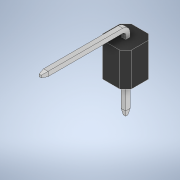
# Autodesk Inventor part: MaleHeaderPin
Saved by Autodesk Inventor 2021 (Build 250183000, 183)
## iProperties
Created: 2020-01-06
Part Number: MaleHeaderPin
Material: Generic
Document SubType Name: Modeling
Designer: ermoz
Density: 1 g/cm^3
Appearance: Default
Mass: 0.0192281 g
Surface Area: 0.622522 cm^2
Volume: 0.0192281 cm^3
Author: ermoz
Autodesk Inventor part; units mm, degrees
ref_plane "YZ Plane" through (0, 0, 0) normal (1, 0, 0) x (0, 1, 0)
ref_plane "XZ Plane" through (0, 0, 0) normal (0, 1, 0) x (-1, 0, 0)
ref_plane "XY Plane" through (0, 0, 0) normal (0, 0, 1) x (1, 0, 0)
sketch "Sketch1" plane through (0, 0, 0) normal (0, 1, 0) x (-1, 0, 0)
  line L0 (-1.27, 1.27) -> (1.27, 1.27)
  line L1 (1.27, 1.27) -> (1.27, -1.27)
  line L2 (1.27, -1.27) -> (-1.27, -1.27)
  line L3 (-1.27, -1.27) -> (-1.27, 1.27)
  line L4 (-1.27, 1.27) -> (1.27, -1.27) construction
  line L5 (1.27, 1.27) -> (-1.27, -1.27) construction
  line L6 (-0.3, 0.3) -> (0.3, 0.3)
  line L7 (0.3, 0.3) -> (0.3, -0.3)
  line L8 (0.3, -0.3) -> (-0.3, -0.3)
  line L9 (-0.3, -0.3) -> (-0.3, 0.3)
  line L10 (-0.3, 0.3) -> (0.3, -0.3) construction
  line L11 (0.3, 0.3) -> (-0.3, -0.3) construction
  point P0 (0, 0)
  dimension "d0" = 2.54
  dimension "d1" = 2.54
  dimension "d2" = 0.6
  dimension "d3" = 0.6
  constraints: 24 end point, 4 midpoint, 4 parallel, 2 horizontal, 2 perpendicular
  measures "d0" distance of L1.end L2.end
  measures "d1" distance of L0.end L1.end
  measures "d2" distance of L7.end L8.end
  measures "d3" distance of L6.end L7.end
extrude "Extrusion1" add sketch "Sketch1" along normal blind 9 and the other way blind 3 contours L6 L7 L8 L9
extrude "Extrusion2" add sketch "Sketch1" along normal blind 3 separate body
sketch "Sketch2" plane through (0, 9, 0) normal (0, 1, 0) x (1, 0, 0)
  line L0 (-0.2, -0.2) -> (0.2, -0.2)
  line L1 (0.2, -0.2) -> (0.2, 0.2)
  line L2 (0.2, 0.2) -> (-0.2, 0.2)
  line L3 (-0.2, 0.2) -> (-0.2, -0.2)
  line L4 (-0.2, -0.2) -> (0.2, 0.2) construction
  line L5 (0.2, -0.2) -> (-0.2, 0.2) construction
  line L6 (-2.0289, -1.4927) -> (2.0289, -1.4927)
  line L7 (2.0289, -1.4927) -> (2.0289, 1.4927)
  line L8 (2.0289, 1.4927) -> (-2.0289, 1.4927)
  line L9 (-2.0289, 1.4927) -> (-2.0289, -1.4927)
  line L10 (-2.0289, -1.4927) -> (2.0289, 1.4927) construction
  line L11 (2.0289, -1.4927) -> (-2.0289, 1.4927) construction
  point P0 (0, 0)
  dimension "d37" = 0.4
  dimension "d38" = 0.4
  constraints: 24 end point, 4 midpoint, 4 parallel, 2 horizontal, 2 perpendicular
  measures "d37" distance of L2.end L1.end
  measures "d38" distance of L1.end L0.end
extrude "Extrusion3" cut sketch "Sketch2" against normal blind 20 bodies 1
sketch "Sketch3" plane through (0, 3, 0) normal (0, 1, 0) x (1, 0, 0)
  line L0 (-0.3, 0.3) -> (0.3, 0.3) projected
  line L1 (-0.3, -0.3) -> (0.3, -0.3)
  line L2 (0.3, -0.3) -> (0.3, 0.3)
  line L3 (0.3, 0.3) -> (-0.3, 0.3)
  line L4 (-0.3, 0.3) -> (-0.3, -0.3)
  line L5 (-0.3, -0.3) -> (0.3, 0.3) construction
  line L6 (0.3, -0.3) -> (-0.3, 0.3) construction
  line L7 (0.2, -0.2) -> (0.2, 0.2) projected
  line L8 (-0.2, -0.2) -> (0.2, -0.2)
  line L9 (0.2, -0.2) -> (0.2, 0.2)
  line L10 (0.2, 0.2) -> (-0.2, 0.2)
  line L11 (-0.2, 0.2) -> (-0.2, -0.2)
  line L12 (-0.2, -0.2) -> (0.2, 0.2) construction
  line L13 (0.2, -0.2) -> (-0.2, 0.2) construction
  point P0 (0, 0)
  constraints: 24 end point, 4 midpoint, 4 parallel, 2 horizontal, 2 perpendicular
extrude "Extrusion4" add sketch "Sketch3" against normal blind 3 bodies 2
chamfer "Chamfer10" distance 0.5 angle 45 4 edges at (1.27, 1.5, -1.27) (-1.27, 1.5, -1.27) (-1.27, 1.5, 1.27) (1.27, 1.5, 1.27)
chamfer "Chamfer11" distance 0.1 distance2 0.5 1 edges at (0.2, 9, 0) measured on face at (-0.0667, 9, -0.0667)
chamfer "Chamfer12" distance 0.1 distance2 0.5 1 edges at (-0.05, 9, 0.2) measured on face at (-0.1, 9, -0.0667)
chamfer "Chamfer13" distance 0.1 distance2 0.5 1 edges at (-0.2, 9, -0.05) measured on face at (-0.1, 9, -0.1)
chamfer "Chamfer14" distance 0.1 distance2 0.5 1 edges at (0, 9, -0.2) measured on face at (0.0333, 9, 0)
chamfer "Chamfer15" distance 0.1 distance2 0.5 1 edges at (-0.2, -3, 0) measured on face at (-0.0667, -3, -0.0667)
chamfer "Chamfer16" distance 0.1 distance2 0.5 1 edges at (0.05, -3, 0.2) measured on face at (0, -3, -0.0667)
chamfer "Chamfer17" distance 0.1 distance2 0.5 1 edges at (0.2, -3, -0.05) measured on face at (0.1, -3, 0)
chamfer "Chamfer18" distance 0.1 distance2 0.5 1 edges at (0, -3, -0.2) measured on face at (0.0333, -3, 0)
sketch "Sketch4" plane through (0.2, 8.5, 0.2) normal (1, 0, 0) x (0, 0, -1)
  line L0 (0.4, 0) -> (0.4, -11) projected
  line L1 (0.4, -4.5) -> (-7.4, -4.5)
  line L2 (-7.4, -4.5) -> (-7.4, -4.9)
  line L3 (-7.4, -4.9) -> (-0.25, -4.9)
  line L4 (0.4, -4.9) -> (0.4, -4.5)
  line L5 (0.1, -11.5) -> (0.3, -11.5) projected
  line L6 (0, 0) -> (0, -11) projected
  line L7 (0, -5.15) -> (0, -5.5)
  arc A0 (0, -5.15) -> (-0.25, -4.9) centre (-0.25, -5.15) ccw
  arc A1 (0.4, -5.15) -> (-0.25, -4.5) centre (-0.25, -5.15) ccw
  line L8 (0, -5.15) -> (0.4, -5.15)
  line L9 (0.4, -4.9) -> (0.4, -5.15)
  line L10 (0.4, -4.5) -> (0, -4.5)
  line L11 (0, -4.5) -> (0, 0.5)
  line L12 (0, 0.5) -> (0.4, 0.5)
  line L13 (0.4, 0.5) -> (0.4, -4.5)
  point P0 (0.2, -8.5)
  point P1 (0, -4.9)
  point P2 (0, -4.55)
  dimension "d70" = 0.4
  dimension "d71" = 7
  dimension "d72" = 7.8
  dimension "d73" = 0.25
  constraints: 22 end point, 7 point on line, 4 parallel, 4 point on circle, 3 perpendicular, 3 tangent, 2 centre point, 2 horizontal, 1 coincident, 1 midpoint, 1 vertical
  measures "d70" distance between parallel lines of L1 L3
  measures "d71" distance between parallel lines of L5 L1
  measures "d72" distance of L1.start L1.end
  measures "d73" radius of A0
extrude "Extrusion5" cut sketch "Sketch4" against normal through all contours L0 L1 L6 L11 L12 L13 | L0 A1 L6 L1 bodies 1
extrude "Extrusion6" add sketch "Sketch4" against normal up to surface (0.4 mm away) contours A1 L6 A0 L3 L2 L1 bodies 1
chamfer "Chamfer19" distance 0.5 distance2 0.1 1 edges at (0.2, 3.8, 7.6) measured on face at (0.2, 3.7333, 2.8333)
chamfer "Chamfer20" distance 0.5 distance2 0.1 1 edges at (-0.2, 3.8, 7.6) measured on face at (-0.2, 3.7333, 2.8333)
chamfer "Chamfer21" distance 0.1 distance2 0.5 1 edges at (0, 4, 7.6) measured on face at (0.0333, 3.8667, 7.6)
chamfer "Chamfer22" distance 0.5 distance2 0.1 1 edges at (0, 3.6, 7.6) measured on face at (-0.0667, 3.6, 2.6667)
body "Solid1"
body "Solid2"
